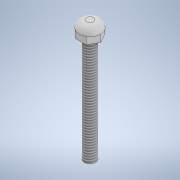
# Autodesk Inventor part: 2in Bolt w Nut
Saved by Autodesk Inventor 2020 (Build 240168000, 168)
## iProperties
Created: 2020-01-08
Part Number: 2in Bolt w Nut
Material: Generic
Document SubType Name: Modeling
Designer: ellio
Density: 1 g/cm^3
Appearance: Default
Author: ellio
Autodesk Inventor part; units mm, degrees
ref_plane "YZ Plane" through (0, 0, 0) normal (1, 0, 0) x (0, 1, 0)
ref_plane "XZ Plane" through (0, 0, 0) normal (0, 1, 0) x (-1, 0, 0)
ref_plane "XY Plane" through (0, 0, 0) normal (0, 0, 1) x (1, 0, 0)
sketch "Sketch1" plane through (0, 0, 0) normal (0, 1, 0) x (-1, 0, 0)
  circle A0 centre (0, 0) radius 4.7625
  dimension "d0" = 9.525
  constraints: 1 centre point, 1 coincident
  measures "d0" diameter of A0
extrude "Extrusion1" add sketch "Sketch1" along normal blind 3.175
fillet "Fillet1" radius 3.175 1 edges at (4.7625, 3.175, 0)
sketch "Sketch2" plane through (0, 0, 0) normal (0, -1, 0) x (1, 0, 0)
  circle A0 centre (0, 0) radius 2.54
  dimension "d4" = 5.08
  constraints: 1 centre point, 1 coincident
  measures "d4" diameter of A0
extrude "Extrusion2" add sketch "Sketch2" along normal blind 50.8
fillet "Fillet2" radius 0.508 1 edges at (-2.54, -50.8, 0)
thread "Thread1" size "12-24 UNC" class "2A" standard "ANSI Unified Screw Threads" full length
sketch "Sketch3" plane through (0, 0, 0) normal (0, -1, 0) x (1, 0, 0)
  circle A0 centre (0, 0) radius 1.5875 projected
  circle A1 centre (0, 0) radius 4.7625 projected
  line L0 (-4.7625, 0) -> (-2.3813, 4.1244)
  line L1 (-2.3813, 4.1244) -> (2.3812, 4.1244)
  line L2 (2.3812, 4.1244) -> (4.7625, 0)
  line L3 (4.7625, 0) -> (2.3813, -4.1244)
  line L4 (2.3813, -4.1244) -> (-2.3812, -4.1244)
  line L5 (-2.3812, -4.1244) -> (-4.7625, 0)
  constraints: 12 end point, 1 coincident, 1 horizontal alignment, 14 other
extrude "Extrusion3" add sketch "Sketch3" along normal blind 3.175 contours L3 L4 L5 L0 L1 L2
body "Solid1"
